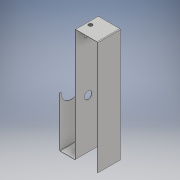
# Autodesk Inventor part: strikkkk
Saved by Autodesk Inventor 2019 (Build 230136000, 136)
## iProperties
Created: 2020-02-20
Part Number: strikkkk
Material: Generic
Document SubType Name: Sheet Metal
Designer: unusualgamer
Density: 1 g/cm^3
Sheet Metal Rule: Default_mm
Appearance: Default
Author: unusualgamer
Autodesk Inventor part; units mm, degrees
ref_plane "YZ Plane" through (0, 0, 0) normal (1, 0, 0) x (0, 1, 0)
ref_plane "XZ Plane" through (0, 0, 0) normal (0, 1, 0) x (-1, 0, 0)
ref_plane "XY Plane" through (0, 0, 0) normal (0, 0, 1) x (1, 0, 0)
sketch "Sketch1" plane through (0, 0, 0) normal (1, 0, 0) x (0, 1, 0)
  line L0 (-78.9055, 475.022) -> (-258.9055, 475.022)
  line L1 (-258.9055, 475.022) -> (-258.9055, 439.022)
  line L2 (-258.9055, 439.022) -> (-78.9055, 439.022)
  line L3 (-78.9055, 439.022) -> (-78.9055, 475.022)
  point P0 (0, 0)
  dimension "d0" = 180
  dimension "d1" = 36
  measures "d0" distance of L2.end L1.end
  measures "d1" distance of L1.end L0.end
extrude "Plate1" add sketch "Sketch1" along normal blind 0.5
sketch "Sketch2" plane through (0.5, -79.4055, 475.022) normal (0, 1, 0) x (1, 0, 0)
  line L0 (0, -36) -> (0, 0)
  line L1 (0, 0) -> (-36, 0)
  line L2 (-36, 0) -> (-36, -36)
  line L3 (-36, -36) -> (0, -36)
  constraints: 6 end point, 1 horizontal, 1 perpendicular, 1 vertical
edge flange "Flange1" height 36 angle 90 thickness 0.5 bend radius 0.5 thickness toward (0, 1, 0) relief tear relief width 0.5 relief depth 0.25 edges at (0.5, -78.9055, 457.022) wall of the first edge with corners at (0.5, -79.4055, 439.022) (0.5, -79.4055, 475.022) (-35.5, -79.4055, 475.022) (-35.5, -79.4055, 439.022)
bend "Bend1"
corner "Corner1"
sketch "Sketch3" plane through (-35, -78.9055, 475.022) normal (-1, 0, 0) x (0, 1, 0)
  line L0 (0, -36) -> (0, 0)
  line L1 (0, 0) -> (-180, 0)
  line L2 (-180, 0) -> (-180, -36)
  line L3 (-180, -36) -> (0, -36)
  constraints: 6 end point, 1 horizontal, 1 perpendicular, 1 vertical
edge flange "Flange2" height 180 angle 90 thickness 0.5 bend radius 0.5 thickness toward (-1, 0, 0) relief tear relief width 0.5 relief depth 0.25 edges at (-35.5, -78.9055, 457.022) wall of the first edge with corners at (-35, -78.9055, 439.022) (-35, -78.9055, 475.022) (-35, -258.9055, 475.022) (-35, -258.9055, 439.022)
bend "Bend2"
corner "Corner2"
sketch "Sketch4" plane through (-35, -258.4055, 439.022) normal (0, -1, 0) x (-1, 0, 0)
  line L0 (0, 36) -> (0, 0)
  line L1 (0, 0) -> (25, 0)
  line L2 (25, 0) -> (25, 36)
  line L3 (25, 36) -> (0, 36)
  constraints: 6 end point, 1 horizontal, 1 perpendicular, 1 vertical
edge flange "Flange3" height 25 angle 90 thickness 0.5 bend radius 0.5 thickness toward (0, -1, 0) relief tear relief width 0.5 relief depth 0.25 edges at (-35, -258.9055, 457.022) wall of the first edge with corners at (-35, -258.4055, 475.022) (-35, -258.4055, 439.022) (-60, -258.4055, 439.022) (-60, -258.4055, 475.022)
bend "Bend3"
corner "Corner3"
sketch "Sketch5" plane through (-59.5, -258.9055, 475.022) normal (-1, 0, 0) x (0, -1, 0)
  line L0 (0, -36) -> (0, 0)
  line L1 (0, 0) -> (-80, 0)
  line L2 (-80, 0) -> (-80, -36)
  line L3 (-80, -36) -> (0, -36)
  constraints: 6 end point, 1 horizontal, 1 perpendicular, 1 vertical
edge flange "Flange4" height 80 angle 90 thickness 0.5 bend radius 0.5 thickness toward (-1, 0, 0) relief tear relief width 0.5 relief depth 0.25 edges at (-60, -258.4055, 457.022) wall of the first edge with corners at (-59.5, -258.9055, 439.022) (-59.5, -258.9055, 475.022) (-59.5, -178.9055, 475.022) (-59.5, -178.9055, 439.022)
bend "Bend4"
corner "Corner4"
sketch "Sketch6" plane through (-59.5, -178.9055, 475.022) normal (1, 0, 0) x (0, 0, -1)
  point P0 (475.022, 178.9055)
  point P1 (18.2971, -1.4985)
hole "Hole1" at (-59.5, -180.404, 456.7249) direction (-1, 0, 0) diameter 33 depth 33 tip angle 118
sketch "Sketch7" plane through (-35, -79.9055, 475.022) normal (1, 0, 0) x (0, 0, -1)
  point P0 (475.022, 79.9055)
  point P1 (20.1704, -99.7704)
hole "Hole2" at (-35, -179.6759, 454.8516) direction (-1, 0, 0) diameter 12.2 depth 0.5 tip angle 118
sketch "Sketch8" plane through (-0.5, -78.9055, 475.022) normal (0, 1, 0) x (1, 0, 0)
  point P0 (0.5, 475.022)
  point P1 (-28.4213, 17.8782)
hole "Hole3" at (-28.9213, -78.9055, 457.1438) direction (0, -1, 0) diameter 6 depth 0.75 tip angle 118
sketch "Sketch9" plane through (-35.5, -79.9055, 439.022) normal (-1, 0, 0) x (0, 0, 1)
  point P0 (-439.022, 79.9055)
  point P1 (19.2457, -16.2545)
hole "Hole4" at (-35.5, -96.16, 458.2677) direction (1, 0, 0) diameter 6 depth 0.5 tip angle 118
equation "\"d55\" = Thickness"
equation "\"d69\" = Thickness"
equation "\"d2\" = Thickness"
equation "\"d3\" = BendReliefWidth"
equation "\"d4\" = BendReliefDepth"
equation "\"d5\" = MinimumRemnant"
equation "\"d6\" = TransitionRadius"
equation "\"d9\" = BendRadius"
equation "\"d10\" = CornerReliefSize"
equation "\"d11\" = GapSize"
equation "\"d12\" = JacobiRadiusSize"
equation "\"d13\" = BendReliefWidth"
equation "\"d14\" = BendReliefDepth"
equation "\"d15\" = MinimumRemnant"
equation "\"d16\" = TransitionRadius"
equation "\"d19\" = BendRadius"
equation "\"d20\" = CornerReliefSize"
equation "\"d21\" = GapSize"
equation "\"d22\" = JacobiRadiusSize"
equation "\"d23\" = BendReliefWidth"
equation "\"d24\" = BendReliefDepth"
equation "\"d25\" = MinimumRemnant"
equation "\"d26\" = TransitionRadius"
equation "\"d29\" = BendRadius"
equation "\"d30\" = CornerReliefSize"
equation "\"d31\" = GapSize"
equation "\"d32\" = JacobiRadiusSize"
equation "\"d33\" = BendReliefWidth"
equation "\"d34\" = BendReliefDepth"
equation "\"d35\" = MinimumRemnant"
equation "\"d36\" = TransitionRadius"
equation "\"d39\" = BendRadius"
equation "\"d40\" = CornerReliefSize"
equation "\"d41\" = GapSize"
equation "\"d42\" = JacobiRadiusSize"
equation "\"BendRadius\" = Thickness"
equation "\"BendReliefWidth\" = Thickness"
equation "\"BendReliefDepth\" = 0.5 * Thickness"
equation "\"CornerReliefSize\" = 4 * Thickness"
equation "\"MinimumRemnant\" = 2 * Thickness"
equation "\"TransitionRadius\" = BendRadius"
equation "\"JacobiRadiusSize\" = BendRadius"
equation "\"GapSize\" = Thickness"
equation "\"Thickness\" = 0.5"
body "Solid1"
